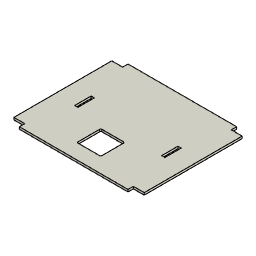
Plate (Autodesk Fusion 360 design; units mm, degrees)
Autodesk Fusion 360 part; units mm, degrees
sketch "Schizzo1" plane through (0, 0, 0) normal (0, 0, 1) x (1, 0, 0)
  line L0 (0, 0) -> (200, 0)
  line L1 (200, 0) -> (200, 200)
  line L2 (200, 200) -> (0, 200)
  line L3 (0, 200) -> (0, 0)
  line L4 (0, 100) -> (200, 100) construction
  line L5 (200, 100) -> (220, 100) construction
  line L6 (0, 100) -> (-20, 100) construction
  line L7 (220, 100) -> (220, 190.15)
  line L8 (220, 190.15) -> (200, 190.15)
  line L9 (220, 100) -> (220, 9.85)
  line L10 (220, 9.85) -> (200, 9.85)
  line L11 (-20, 100) -> (-20, 190.15)
  line L12 (-20, 190.15) -> (0, 190.15)
  line L13 (-20, 100) -> (-20, 9.85)
  line L14 (-20, 9.85) -> (0, 9.85)
  line L15 (0, 190.15) -> (200, 190.15) construction
  line L16 (200, 9.85) -> (0, 9.85) construction
  line L17 (0, 49.85) -> (200, 49.85) construction
  line L18 (122, 71.85) -> (78, 71.85)
  line L19 (78, 71.85) -> (78, 27.85)
  line L20 (78, 27.85) -> (122, 27.85)
  line L21 (122, 27.85) -> (122, 71.85)
  line L22 (122, 71.85) -> (78, 27.85) construction
  line L23 (78, 71.85) -> (122, 27.85) construction
  line L24 (23, 115) -> (17, 115)
  line L25 (17, 115) -> (17, 85)
  line L26 (17, 85) -> (23, 85)
  line L27 (23, 85) -> (23, 115)
  line L28 (23, 115) -> (17, 85) construction
  line L29 (17, 115) -> (23, 85) construction
  line L30 (183, 115) -> (177, 115)
  line L31 (177, 115) -> (177, 85)
  line L32 (177, 85) -> (183, 85)
  line L33 (183, 85) -> (183, 115)
  line L34 (183, 115) -> (177, 85) construction
  line L35 (177, 115) -> (183, 85) construction
  point P0 (100, 49.85)
  point P1 (20, 100)
  point P2 (180, 100)
  dimension "d1" = 200
  dimension "d2" = 200
  dimension "d3" = 180.3
  dimension "d4" = 20
  dimension "d10" = 40
  dimension "d11" = 44
  dimension "d12" = 44
  dimension "d15" = 20
  dimension "d16" = 20
  dimension "d17" = 30
  dimension "d18" = 6
  dimension "d19" = 6
  dimension "d20" = 30
  constraint horizontal L0
  constraint vertical L1
  constraint horizontal L2
  constraint vertical L3
  constraint coincident L0.start L3.end
  constraint midpoint L3 L4.start
  constraint midpoint L1 L4.end
  constraint perpendicular L1 L5
  constraint perpendicular L3 L6
  constraint perpendicular L5 L7
  constraint coincident L1 L8.end
  constraint perpendicular L1 L8
  constraint perpendicular L8 L9
  constraint coincident L1 L10.end
  constraint perpendicular L1 L10
  constraint perpendicular L6 L11
  constraint coincident L3 L12.end
  constraint perpendicular L3 L12
  constraint perpendicular L6 L13
  constraint coincident L3 L14.end
  constraint perpendicular L3 L14
  constraint equal L11 L13
  constraint equal L7 L9
  constraint equal L7 L11
  constraint equal L10 L14
  constraint coincident L3 L17.start
  constraint coincident L1 L17.end
  constraint perpendicular L1 L17
  constraint horizontal L18
  constraint perpendicular L18 L19
  constraint parallel L18 L20
  constraint parallel L19 L21
  constraint coincident L22 P0
  constraint coincident L23 P0
  constraint midpoint L17 P0
  constraint horizontal L24
  constraint perpendicular L24 L25
  constraint parallel L24 L26
  constraint parallel L25 L27
  constraint coincident L28 P1
  constraint coincident L29 P1
  constraint coincident L4 P1
  constraint horizontal L30
  constraint perpendicular L30 L31
  constraint parallel L30 L32
  constraint parallel L31 L33
  constraint coincident L34 P2
  constraint coincident L35 P2
  constraint coincident L4 P2
  measures "d1" distance of L0.start L2.end
  measures "d2" distance of L0.start L0.end
  measures "d3" distance of L12 L14
  measures "d4" distance of L13.end L14.end
  measures "d10" distance of L16 L17
  measures "d11" distance of L19.end L20.end
  measures "d12" distance of L18.end L19.end
  measures "d15" distance of L3 P1
  measures "d16" distance of L1 P2
  measures "d17" distance of L24.start L26.end
  measures "d18" distance of L24.start L24.end
  measures "d19" distance of L30.start L30.end
  measures "d20" distance of L30.end L31.end
extrude "Estrusione1" add sketch "Schizzo1" along normal blind 4
fillet "Raccordo1" radius 2 4 edges at (122, 27.85, 2) (78, 27.85, 2) (78, 71.85, 2) (122, 71.85, 2)
component "Component" placed x (1, 0, 0) y (0, 1, 0) z (0, 0, 1) at (0, 0, 0)
equation "d3 = 180 mm + 2 * t"
equation "h = 4 mm"
equation "t = 0.15 mm"
equation "d7 = h"
